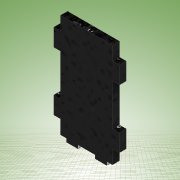
# Autodesk Inventor part: Caja_CaraFrontal
Saved by Autodesk Inventor 2022 (Build 260153000, 153)
## iProperties
Created: 2022-03-02
Part Number: Caja_CaraFrontal
Material: Genérico
Document SubType Name: Modeling
Designer: Marco
Density: 1 g/cm^3
Appearance: Valor por defecto
Author: Marco
Autodesk Inventor part; units mm, degrees
ref_plane "YZ Plane" through (0, 0, 0) normal (1, 0, 0) x (0, 1, 0)
ref_plane "XZ Plane" through (0, 0, 0) normal (0, 1, 0) x (-1, 0, 0)
ref_plane "XY Plane" through (0, 0, 0) normal (0, 0, 1) x (1, 0, 0)
sketch "Boceto1" plane through (0, 0, 0) normal (0, 0, 1) x (1, 0, 0)
  line L0 (0, 0) -> (45, 0)
  line L1 (45, 0) -> (45, 90)
  line L2 (45, 90) -> (0, 90)
  line L3 (0, 90) -> (0, 0)
  line L4 (45, 78) -> (51, 78)
  line L5 (51, 78) -> (51, 63)
  line L6 (51, 63) -> (45, 63)
  line L7 (45, 63) -> (45, 78)
  line L8 (45, 45) -> (0, 45)
  line L9 (45, 12) -> (51, 12)
  line L10 (51, 12) -> (51, 27)
  line L11 (51, 27) -> (45, 27)
  line L12 (45, 27) -> (45, 12)
  line L13 (22.5, 90) -> (22.5, 45)
  line L14 (0, 78) -> (-6, 78)
  line L15 (-6, 78) -> (-6, 63)
  line L16 (-6, 63) -> (0, 63)
  line L17 (0, 63) -> (0, 78)
  line L18 (0, 12) -> (-6, 12)
  line L19 (-6, 12) -> (-6, 27)
  line L20 (-6, 27) -> (0, 27)
  line L21 (0, 27) -> (0, 12)
  dimension "d0" = 45
  dimension "d1" = 90
  dimension "d2" = 6
  dimension "d3" = 15
  dimension "d4" = 12
  constraints: 44 end point, 12 symmetric about line, 4 midpoint, 4 parallel, 2 horizontal, 2 perpendicular, 1 point on line
  measures "d0" distance of L2.end L1.end
  measures "d1" distance of L2.end L0.start
  measures "d2" distance of L5.end L6.end
  measures "d3" distance of L4.end L5.end
  measures "d4" distance of L4.start L1.end
extrude "Extrusión1" add sketch "Boceto1" along normal blind 6
sketch "Boceto2" plane through (0, 0, 0) normal (0, -1, 0) x (1, 0, 0)
  line L0 (0, 6) -> (45, 6) projected
  line L1 (0, 0) -> (45, 0) projected
  line L2 (5, 6) -> (15, 6)
  line L3 (15, 6) -> (15, 0)
  line L4 (15, 0) -> (5, 0)
  line L5 (5, 0) -> (5, 6)
  line L6 (22.5, 0) -> (22.5, 6)
  line L7 (40, 6) -> (30, 6)
  line L8 (30, 6) -> (30, 0)
  line L9 (30, 0) -> (40, 0)
  line L10 (40, 0) -> (40, 6)
  point P0 (5, 0)
  dimension "d7" = 10
  dimension "d8" = 5
  constraints: 18 end point, 4 symmetric about line, 2 midpoint, 2 parallel, 2 point on line, 1 horizontal, 1 perpendicular
  measures "d7" distance of L3.end L4.end
  measures "d8" distance of L1.start L4.end
extrude "Extrusión2" add sketch "Boceto2" along normal blind 3 contours L0 L3 L1 L5 | L0 L10 L1 L8
